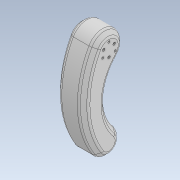
# Autodesk Inventor part: thigh_link
Saved by Autodesk Inventor 2020 (Build 240168000, 168)
## iProperties
Created: 2020-12-22
Part Number: thigh_link
Material: Generic
Document SubType Name: Modeling
Designer: DELL
Density: 1 g/cm^3
Appearance: Default
Author: DELL
Autodesk Inventor part; units mm, degrees
ref_plane "YZ Plane" through (0, 0, 0) normal (1, 0, 0) x (0, 1, 0)
ref_plane "XZ Plane" through (0, 0, 0) normal (0, 1, 0) x (-1, 0, 0)
ref_plane "XY Plane" through (0, 0, 0) normal (0, 0, 1) x (1, 0, 0)
sketch "Sketch1" plane through (0, 0, 0) normal (1, 0, 0) x (0, 1, 0)
  circle A0 centre (0, 0) radius 11.5 construction
  line L0 (0, 0) -> (-130, 0) construction
  circle A1 centre (11.5, 0) radius 1.65
  circle A2 centre (-5.75, 9.9593) radius 1.65
  circle A3 centre (-5.75, -9.9593) radius 1.65
  line L1 (0, 0) -> (-5.75, 9.9593) construction
  line L2 (0, 0) -> (-5.75, -9.9593) construction
  line L3 (0, 11.5) -> (0, -11.5) construction
  circle A4 centre (0, 0) radius 9.715 construction
  circle A5 centre (-9.715, 0) radius 2
  circle A6 centre (4.8575, 8.4134) radius 2
  circle A7 centre (4.8575, -8.4134) radius 2
  line L4 (0, 0) -> (5.75, 9.9593) construction
  line L5 (0, 0) -> (5.75, -9.9593) construction
  circle A8 centre (0, 0) radius 25
  circle A9 centre (-130, 0) radius 20
  circle A10 centre (11.5, 0) radius 2.75
  circle A11 centre (-5.75, 9.9593) radius 2.75
  circle A12 centre (-5.75, -9.9593) radius 2.75
  circle A13 centre (-60.0962, -109.6059) radius 150
  circle A14 centre (-68.75, -72.6184) radius 75
  point P0 (-65, 0)
  point P1 (13, 21.3542)
  point P2 (-13, -21.3542)
  point P3 (-117.1053, -15.2881)
  point P4 (-17.1875, -18.1546)
  point P5 (12.0192, 21.9212)
  point P6 (-140.7544, 16.8624)
  dimension "d0" = 23
  dimension "d1" = 130
  dimension "d2" = 3.3
  dimension "d3" = 30
  dimension "d4" = 30
  dimension "d5" = 19.43
  dimension "d6" = 4
  dimension "d7" = 30
  dimension "d8" = 50
  dimension "d12" = 5.5
  dimension "d25" = 40
  dimension "d26" = 150
  dimension "d27" = 300
  constraints: 14 centre point, 12 end point, 7 coincident, 6 equal radius, 5 point on circle, 4 tangent, 3 midpoint, 3 point on line, 2 horizontal alignment, 1 horizontal, 1 vertical, 10 other
  measures "d1" distance of L0.end point (0, 0)
  measures "d2" diameter of A1
  measures "d3" angle of L3 L1
  measures "d4" angle of L3 L2
  measures "d5" diameter of A4
  measures "d6" diameter of A6
  measures "d7" angle of L3 L4
  measures "d8" diameter of A8
  measures "d12" diameter of A10
  measures "d25" diameter of A9
  measures "d26" diameter of A14
  measures "d27" diameter of A13
extrude "Extrusion1" add sketch "Sketch1" against normal mid plane 45 contours A5 | A6 | A7 | A8 | A8 A14 A9 A13 | A9 | A10 | A11 | A12 picked at (-97.8967, 15.2193)
extrude "Extrusion2" cut sketch "Sketch1" along normal blind 35 from surface at -22.5 contours A10 | A11 | A12
extrude "Extrusion3" cut sketch "Sketch1" against normal blind 5 from surface at 22.5 contours A5 | A6 | A7
chamfer "Chamfer1" distance 8 angle 45 2 edges at (22.5, 20.2038, -14.7243) (22.5, -146.1108, -11.8508)
chamfer "Chamfer2" distance 8 angle 45 2 edges at (-22.5, 20.2038, -14.7243) (-22.5, -146.1108, -11.8508)
fillet "Fillet1" radius 5 8 edges at (-14.5, -146.1108, -11.8508) (-14.5, 20.2038, -14.7243) (-22.5, -139.6665, -7.1105) (-22.5, 13.7386, -10.0125) (14.5, -146.1108, -11.8508) (14.5, 20.2038, -14.7243) (22.5, -139.6665, -7.1105) (22.5, 13.7386, -10.0125)
equation "\"d1\" = shank_length"
equation "\"shank_length\" = 130"
body "Solid1"
